Autodesk Fusion 360 part; units mm, degrees
(part 4 of 5)
sketch "Sketch10" plane through (0, 0, 4.8) normal (0, 0, 1) x (-1, 0, 0)
  circle A0 centre (0, 0) radius 3
  line L0 (57.7941, -61.1213) -> (57.7941, -86.8787)
  arc A1 (55.6728, -89) -> (57.7941, -86.8787) centre (56.7335, -87.9393) ccw
  line L1 (55.6728, -89) -> (53.2941, -89)
  line L2 (53.2941, -89) -> (53.2941, -89.8787)
  arc A2 (51.1728, -92) -> (53.2941, -89.8787) centre (52.2335, -90.9393) ccw
  line L3 (51.1728, -92) -> (18.4155, -92)
  arc A3 (16.2941, -89.8787) -> (18.4155, -92) centre (17.3548, -90.9393) ccw
  line L4 (16.2941, -89.8787) -> (16.2941, -89)
  line L5 (16.2941, -89) -> (13.9155, -89)
  arc A4 (11.7941, -86.8787) -> (13.9155, -89) centre (12.8548, -87.9393) ccw
  line L6 (11.7941, -86.8787) -> (11.7941, -61.1213)
  arc A5 (13.9155, -59) -> (11.7941, -61.1213) centre (12.8548, -60.0607) ccw
  line L7 (13.9155, -59) -> (16.2941, -59)
  line L8 (16.2941, -59) -> (16.2941, -58.1213)
  arc A6 (18.4155, -56) -> (16.2941, -58.1213) centre (17.3548, -57.0607) ccw
  line L9 (18.4155, -56) -> (51.1728, -56)
  arc A7 (53.2941, -58.1213) -> (51.1728, -56) centre (52.2335, -57.0607) ccw
  line L10 (53.2941, -58.1213) -> (53.2941, -59)
  line L11 (53.2941, -59) -> (55.6728, -59)
  arc A8 (57.7941, -61.1213) -> (55.6728, -59) centre (56.7335, -60.0607) ccw
  line L12 (51.1728, 56) -> (18.4155, 56)
  arc A9 (16.2941, 58.1213) -> (18.4155, 56) centre (17.3548, 57.0607) ccw
  line L13 (16.2941, 58.1213) -> (16.2941, 59)
  line L14 (16.2941, 59) -> (13.9155, 59)
  arc A10 (11.7941, 61.1213) -> (13.9155, 59) centre (12.8548, 60.0607) ccw
  line L15 (11.7941, 61.1213) -> (11.7941, 86.8787)
  arc A11 (13.9155, 89) -> (11.7941, 86.8787) centre (12.8548, 87.9393) ccw
  line L16 (13.9155, 89) -> (16.2941, 89)
  line L17 (16.2941, 89) -> (16.2941, 89.8787)
  arc A12 (18.4155, 92) -> (16.2941, 89.8787) centre (17.3548, 90.9393) ccw
  line L18 (18.4155, 92) -> (51.1728, 92)
  arc A13 (53.2941, 89.8787) -> (51.1728, 92) centre (52.2335, 90.9393) ccw
  line L19 (53.2941, 89.8787) -> (53.2941, 89)
  line L20 (53.2941, 89) -> (55.6728, 89)
  arc A14 (57.7941, 86.8787) -> (55.6728, 89) centre (56.7335, 87.9393) ccw
  line L21 (57.7941, 86.8787) -> (57.7941, 61.1213)
  arc A15 (55.6728, 59) -> (57.7941, 61.1213) centre (56.7335, 60.0607) ccw
  line L22 (55.6728, 59) -> (53.2941, 59)
  line L23 (53.2941, 59) -> (53.2941, 58.1213)
  arc A16 (51.1728, 56) -> (53.2941, 58.1213) centre (52.2335, 57.0607) ccw
  arc A17 (65.7941, 74.3) -> (67.2941, 72.8) centre (67.2941, 74.3) ccw
  line L24 (65.7941, 74.3) -> (65.7941, 100.26)
  arc A18 (68.1301, 101.5054) -> (65.7941, 100.26) centre (67.2941, 100.26) ccw
  arc A19 (96.3668, 75.223) -> (68.1301, 101.5054) centre (0, 0) ccw
  arc A20 (95.1844, 72.8) -> (96.3668, 75.223) centre (95.1844, 74.3) ccw
  line L25 (95.1844, 72.8) -> (67.2941, 72.8)
  arc A21 (65.7941, -100.26) -> (68.1301, -101.5054) centre (67.2941, -100.26) ccw
  line L26 (65.7941, -100.26) -> (65.7941, -74.3)
  arc A22 (67.2941, -72.8) -> (65.7941, -74.3) centre (67.2941, -74.3) ccw
  line L27 (67.2941, -72.8) -> (95.1844, -72.8)
  arc A23 (96.3668, -75.223) -> (95.1844, -72.8) centre (95.1844, -74.3) ccw
  arc A24 (68.1301, -101.5054) -> (96.3668, -75.223) centre (0, 0) ccw
  circle A25 centre (64.2941, -62.4) radius 1.5
  circle A26 centre (64.2941, 62.4) radius 1.5
  circle A27 centre (97.2941, -62.4) radius 1.5
  circle A28 centre (97.2941, 62.4) radius 1.5
  line L28 (15.4941, 111.4) -> (41.8941, 111.4)
  arc A29 (45.5941, 107.7) -> (41.8941, 111.4) centre (41.8941, 107.7) ccw
  line L29 (45.5941, 107.7) -> (45.5941, 100.7)
  arc A30 (41.8941, 97) -> (45.5941, 100.7) centre (41.8941, 100.7) ccw
  line L30 (41.8941, 97) -> (15.4941, 97)
  arc A31 (11.7941, 100.7) -> (15.4941, 97) centre (15.4941, 100.7) ccw
  line L31 (11.7941, 100.7) -> (11.7941, 107.7)
  arc A32 (15.4941, 111.4) -> (11.7941, 107.7) centre (15.4941, 107.7) ccw
  line L32 (15.4941, -97) -> (41.8941, -97)
  arc A33 (45.5941, -100.7) -> (41.8941, -97) centre (41.8941, -100.7) ccw
  line L33 (45.5941, -100.7) -> (45.5941, -107.7)
  arc A34 (41.8941, -111.4) -> (45.5941, -107.7) centre (41.8941, -107.7) ccw
  line L34 (41.8941, -111.4) -> (15.4941, -111.4)
  arc A35 (11.7941, -107.7) -> (15.4941, -111.4) centre (15.4941, -107.7) ccw
  line L35 (11.7941, -107.7) -> (11.7941, -100.7)
  arc A36 (15.4941, -97) -> (11.7941, -100.7) centre (15.4941, -100.7) ccw
  arc A37 (94.6728, -10) -> (96.7941, -7.8787) centre (95.7335, -8.9393) ccw
  line L36 (94.6728, -10) -> (94.1155, -10)
  arc A38 (91.9941, -7.8787) -> (94.1155, -10) centre (93.0548, -8.9393) ccw
  line L37 (91.9941, -7.8787) -> (91.9941, 7.8787)
  arc A39 (94.1155, 10) -> (91.9941, 7.8787) centre (93.0548, 8.9393) ccw
  line L38 (94.1155, 10) -> (94.6728, 10)
  arc A40 (96.7941, 7.8787) -> (94.6728, 10) centre (95.7335, 8.9393) ccw
  line L39 (96.7941, 7.8787) -> (96.7941, -7.8787)
  circle A41 centre (-94.9024, 87.3758) radius 1.5
  circle A42 centre (123.1209, -38.5) radius 1.5
  circle A43 centre (45.4941, 42.5) radius 1.5
  circle A44 centre (45.4941, -42.5) radius 1.5
  circle A45 centre (123.1209, 38.5) radius 1.5
  circle A46 centre (64.5, -111.7173) radius 1.5
  circle A47 centre (-28.2185, 125.8758) radius 1.5
  circle A48 centre (-94.9024, -87.3758) radius 1.5
  circle A49 centre (-28.2185, -125.8758) radius 1.5
  circle A50 centre (64.5, 111.7173) radius 1.5
  circle A51 centre (-123.5112, -37.2289) radius 1.5
  circle A52 centre (-123.5112, 37.2289) radius 1.5
  arc A53 (-55.2202, 79.8868) -> (-55.9967, 76.9891) centre (-55.6084, 78.438) ccw
  line L40 (-55.2202, 79.8868) -> (-41.5739, 87.7655)
  arc A54 (-38.6762, 86.9891) -> (-41.5739, 87.7655) centre (-40.125, 87.3773) ccw
  line L41 (-38.6762, 86.9891) -> (-38.3975, 86.5064)
  arc A55 (-39.1739, 83.6086) -> (-38.3975, 86.5064) centre (-38.7857, 85.0575) ccw
  line L42 (-39.1739, 83.6086) -> (-52.8202, 75.7299)
  arc A56 (-55.718, 76.5064) -> (-52.8202, 75.7299) centre (-54.2691, 76.1181) ccw
  line L43 (-55.718, 76.5064) -> (-55.9967, 76.9891)
  arc A57 (-11.2762, 39.5309) -> (-14.1739, 40.3073) centre (-12.725, 39.9191) ccw
  line L44 (-11.2762, 39.5309) -> (-10.9975, 39.0482)
  arc A58 (-11.7739, 36.1504) -> (-10.9975, 39.0482) centre (-11.3857, 37.5993) ccw
  line L45 (-11.7739, 36.1504) -> (-25.4202, 28.2717)
  arc A59 (-28.318, 29.0482) -> (-25.4202, 28.2717) centre (-26.8691, 28.66) ccw
  line L46 (-28.318, 29.0482) -> (-28.5967, 29.5309)
  arc A60 (-27.8202, 32.4286) -> (-28.5967, 29.5309) centre (-28.2084, 30.9798) ccw
  line L47 (-27.8202, 32.4286) -> (-14.1739, 40.3073)
  arc A61 (-10.9975, -39.0482) -> (-11.7739, -36.1504) centre (-11.3857, -37.5993) ccw
  line L48 (-10.9975, -39.0482) -> (-11.2762, -39.5309)
  arc A62 (-14.1739, -40.3073) -> (-11.2762, -39.5309) centre (-12.725, -39.9191) ccw
  line L49 (-14.1739, -40.3073) -> (-27.8202, -32.4286)
  arc A63 (-28.5967, -29.5309) -> (-27.8202, -32.4286) centre (-28.2084, -30.9798) ccw
  line L50 (-28.5967, -29.5309) -> (-28.318, -29.0482)
  arc A64 (-25.4202, -28.2717) -> (-28.318, -29.0482) centre (-26.8691, -28.66) ccw
  line L51 (-25.4202, -28.2717) -> (-11.7739, -36.1504)
  arc A65 (-52.8202, -75.7299) -> (-55.718, -76.5064) centre (-54.2691, -76.1181) ccw
  line L52 (-52.8202, -75.7299) -> (-39.1739, -83.6086)
  arc A66 (-38.3975, -86.5064) -> (-39.1739, -83.6086) centre (-38.7857, -85.0575) ccw
  line L53 (-38.3975, -86.5064) -> (-38.6762, -86.9891)
  arc A67 (-41.5739, -87.7655) -> (-38.6762, -86.9891) centre (-40.125, -87.3773) ccw
  line L54 (-41.5739, -87.7655) -> (-55.2202, -79.8868)
  arc A68 (-55.9967, -76.9891) -> (-55.2202, -79.8868) centre (-55.6084, -78.438) ccw
  line L55 (-55.9967, -76.9891) -> (-55.718, -76.5064)
  arc A69 (39.8728, -10) -> (41.9941, -7.8787) centre (40.9335, -8.9393) ccw
  line L56 (39.8728, -10) -> (39.3155, -10)
  arc A70 (37.1941, -7.8787) -> (39.3155, -10) centre (38.2548, -8.9393) ccw
  line L57 (37.1941, -7.8787) -> (37.1941, 7.8787)
  arc A71 (39.3155, 10) -> (37.1941, 7.8787) centre (38.2548, 8.9393) ccw
  line L58 (39.3155, 10) -> (39.8728, 10)
  arc A72 (41.9941, 7.8787) -> (39.8728, 10) centre (40.9335, 8.9393) ccw
  line L59 (41.9941, 7.8787) -> (41.9941, -7.8787)
  line L60 (-42.1213, -25.5) -> (-109.5263, -25.5)
  arc A73 (-109.5263, -25.5) -> (-110.7763, -25.8349) centre (-109.5263, -28) ccw
  line L61 (-110.7763, -25.8349) -> (-125.9451, -34.5927)
  arc A74 (-125.9451, -34.5927) -> (-127.0931, -37.4646) centre (-124.6951, -36.7577) ccw
  arc A75 (-127.0931, -37.4646) -> (-89.0244, -98.1371) centre (0, 0) ccw
  arc A76 (-89.0244, -98.1371) -> (-85.1797, -97.5355) centre (-87.3447, -96.2855) ccw
  line L62 (-85.1797, -97.5355) -> (-74.6084, -79.2255)
  arc A77 (-71.7106, -78.449) -> (-74.6084, -79.2255) centre (-73.1595, -78.8372) ccw
  line L63 (-71.7106, -78.449) -> (-32.0836, -101.3277)
  arc A78 (-31.3071, -104.2255) -> (-32.0836, -101.3277) centre (-31.6953, -102.7766) ccw
  line L64 (-31.3071, -104.2255) -> (-41.8784, -122.5355)
  arc A79 (-41.8784, -122.5355) -> (-40.477, -126.166) centre (-39.7133, -123.7855) ccw
  arc A80 (-40.477, -126.166) -> (129.5015, -28.0288) centre (0, 0) ccw
  arc A81 (129.5015, -28.0288) -> (127.0581, -25) centre (127.0581, -27.5) ccw
  line L65 (127.0581, -25) -> (105.9155, -25)
  arc A82 (103.7941, -22.8787) -> (105.9155, -25) centre (104.8548, -23.9393) ccw
  line L66 (103.7941, -22.8787) -> (103.7941, 22.8787)
  arc A83 (105.9155, 25) -> (103.7941, 22.8787) centre (104.8548, 23.9393) ccw
  line L67 (105.9155, 25) -> (127.0581, 25)
  arc A84 (127.0581, 25) -> (129.5015, 28.0288) centre (127.0581, 27.5) ccw
  arc A85 (129.5015, 28.0288) -> (-40.477, 126.166) centre (0, 0) ccw
  arc A86 (-40.477, 126.166) -> (-41.8784, 122.5355) centre (-39.7133, 123.7855) ccw
  line L68 (-41.8784, 122.5355) -> (-31.3071, 104.2255)
  arc A87 (-32.0836, 101.3277) -> (-31.3071, 104.2255) centre (-31.6953, 102.7766) ccw
  line L69 (-32.0836, 101.3277) -> (-71.7106, 78.449)
  arc A88 (-74.6084, 79.2255) -> (-71.7106, 78.449) centre (-73.1595, 78.8372) ccw
  line L70 (-74.6084, 79.2255) -> (-85.1797, 97.5355)
  arc A89 (-85.1797, 97.5355) -> (-89.0244, 98.1371) centre (-87.3447, 96.2855) ccw
  arc A90 (-89.0244, 98.1371) -> (-127.0931, 37.4646) centre (0, 0) ccw
  arc A91 (-127.0931, 37.4646) -> (-125.9451, 34.5927) centre (-124.6951, 36.7577) ccw
  line L71 (-125.9451, 34.5927) -> (-110.7763, 25.8349)
  arc A92 (-110.7763, 25.8349) -> (-109.5263, 25.5) centre (-109.5263, 28) ccw
  line L72 (-109.5263, 25.5) -> (-42.1213, 25.5)
  arc A93 (-40, 23.3787) -> (-42.1213, 25.5) centre (-41.0607, 24.4393) ccw
  line L73 (-40, 23.3787) -> (-40, 20.8)
  arc A94 (-40, 20.8) -> (-37.5, 18.3) centre (-37.5, 20.8) ccw
  line L74 (-37.5, 18.3) -> (-34.1213, 18.3)
  arc A95 (-32, 16.1787) -> (-34.1213, 18.3) centre (-33.0607, 17.2393) ccw
  line L75 (-32, 16.1787) -> (-32, -16.1787)
  arc A96 (-34.1213, -18.3) -> (-32, -16.1787) centre (-33.0607, -17.2393) ccw
  line L76 (-34.1213, -18.3) -> (-37.5, -18.3)
  arc A97 (-37.5, -18.3) -> (-40, -20.8) centre (-37.5, -20.8) ccw
  line L77 (-40, -20.8) -> (-40, -23.3787)
  arc A98 (-42.1213, -25.5) -> (-40, -23.3787) centre (-41.0607, -24.4393) ccw
  line L78 (-42.1213, 25.5) -> (-109.5263, 25.5)
  line L79 (-42.1213, -25.5) -> (-109.5263, -25.5)
  arc A99 (-127.0931, -37.4646) -> (-89.0244, -98.1371) centre (0, 0) ccw
  arc A100 (-89.0244, 98.1371) -> (-127.0931, 37.4646) centre (0, 0) ccw
  line L80 (-25.6319, 7.5958) -> (-67.8319, 80.6884)
  line L81 (-25.6319, -7.5958) -> (-67.8319, -80.6884)
  circle A101 centre (-53.2894, 35.5) radius 1.5
  circle A102 centre (-100, 35.5) radius 1.5
  line L82 (-130.0231, 25.5) -> (-40, 25.5)
  line L83 (-100, 25.5) -> (-100, -25.5) construction
  line L84 (-40, 25.5) -> (-40, -25.5) construction
  line L85 (-100, 25.5) -> (-100, 35.5) construction
  circle A103 centre (-53.2894, -35.5) radius 1.5
  circle A104 centre (-100, -35.5) radius 1.5
  line L86 (-100, -25.5) -> (-100, -35.5) construction
  line L87 (-103, 28.5) -> (-103, 35.5)
  line L88 (-100, 38.5) -> (-48.1666, 38.5)
  line L89 (0, 0) -> (-44.1633, 38.5) construction
  line L90 (-47.1809, 41.1307) -> (-97.2023, 84.7376)
  line L91 (-85.1797, 97.5355) -> (-74.6084, 79.2255)
  line L92 (-103, 25.5) -> (-103, 28.5) construction
  arc A105 (-100, 25.5) -> (-103, 28.5) centre (-100, 28.5) ccw construction
  arc A106 (-103, 28.5) -> (-100, 25.5) centre (-100, 28.5) ccw
  arc A107 (-48.1666, 38.5) -> (-47.1809, 41.1307) centre (-48.1666, 40) ccw
  arc A108 (-100, 38.5) -> (-103, 35.5) centre (-100, 35.5) ccw
  arc A109 (-40.477, 126.166) -> (-40.477, -126.166) centre (0, 0) ccw
  line L93 (-97.2023, 84.7376) -> (-99.8764, 87.0687) construction
  arc A110 (-97.2023, 84.7376) -> (-97.4773, 89.7465) centre (-94.9024, 87.3758) ccw construction
  arc A111 (-97.4773, 89.7465) -> (-97.2023, 84.7376) centre (-94.9024, 87.3758) ccw
  line L94 (0, 0) -> (-44.1633, -38.5) construction
  line L95 (-48.1666, -38.5) -> (-100, -38.5)
  line L96 (-103, -35.5) -> (-103, -28.5)
  line L97 (-47.1809, -41.1307) -> (-97.2023, -84.7376)
  arc A112 (-47.1809, -41.1307) -> (-48.1666, -38.5) centre (-48.1666, -40) ccw
  arc A113 (-103, -35.5) -> (-100, -38.5) centre (-100, -35.5) ccw
  arc A114 (-97.4773, -89.7465) -> (-97.2023, -84.7376) centre (-94.9024, -87.3758) ccw construction
  arc A115 (-97.2023, -84.7376) -> (-97.4773, -89.7465) centre (-94.9024, -87.3758) ccw
  line L98 (-97.2023, -84.7376) -> (-99.8764, -87.0687) construction
  line L99 (-40, -25.5) -> (-130.0231, -25.5)
  arc A116 (-100, -31.5) -> (-100, -25.5) centre (-100, -28.5) ccw construction
  arc A117 (-100, -25.5) -> (-103, -28.5) centre (-100, -28.5) ccw
  arc A118 (-103, -28.5) -> (-100, -31.5) centre (-100, -28.5) ccw construction
  line L100 (-103, -28.5) -> (-103, -25.5) construction
  point P0 (-94.9024, 87.3758)
  point P1 (-94.9024, -87.3758)
  dimension "d371" = 3
  dimension "d372" = 3
  dimension "d373" = 10
  dimension "d374" = 10
  dimension "d375" = 10
  dimension "d376" = 60
  dimension "d377" = 3
  dimension "d378" = 3
  dimension "d379" = 10
  dimension "d380" = 10
  dimension "d381" = 10
  dimension "d383" = 3
  dimension "d384" = 3
  dimension "d385" = 6
  dimension "d386" = 1.5
  dimension "d387" = 3
  dimension "d388" = 7
  dimension "d389" = 3.5
  dimension "d390" = 3
  dimension "d391" = 3
  dimension "d392" = 3.5
  dimension "d393" = 1.5
  dimension "d394" = 3
  dimension "d395" = 3
  constraint coincident L82 L83.start
  constraint coincident L79 L83.end
  constraint perpendicular L79 L83
  constraint coincident A102.centre L85.end
  constraint vertical L85
  constraint coincident A104.centre L86.end
  constraint vertical L86
  constraint coincident L82 L92.start
  constraint perpendicular L82 L87
  constraint perpendicular L85 L88
  constraint coincident A0.centre A19.centre
  constraint coincident A100 L93.end
  constraint parallel L89 L90
  constraint tangent L87 A105
  constraint tangent L82 A105
  constraint perpendicular L82 L92
  constraint coincident L72 L83.start
  constraint concentric A105 A106
  constraint coincident L89.end L90
  constraint coincident L89.end L88
  constraint tangent L90 A107
  constraint tangent L88 A107
  constraint tangent L88 A108
  constraint tangent L87 A108
  constraint tangent L90 A110
  constraint tangent A109 A110
  constraint parallel L89 L93
  constraint coincident A90 A110.end
  constraint concentric A110 A111
  constraint coincident A99 L98.end
  constraint horizontal L95
  constraint coincident L79 L100.end
  constraint perpendicular L79 L96
  constraint coincident L94.end L97
  constraint coincident L94.end L95
  constraint tangent L97 A112
  constraint tangent L95 A112
  constraint tangent L95 A113
  constraint tangent L96 A113
  constraint coincident P1 A48.centre
  constraint tangent L97 A114
  constraint coincident A75 A114.start
  constraint concentric A114 A115
  constraint coincident L94.end L98
  constraint tangent L96 A116
  constraint tangent L99 A116
  constraint coincident L60 L83.end
  constraint concentric A116 A117
  constraint coincident L86 A116.start
  constraint concentric A116 A118
  constraint perpendicular L79 L100
  measures "d371" diameter of A101
  measures "d372" diameter of A102
  measures "d373" distance of L80 A101.centre
  measures "d374" distance of A101.centre L82
  measures "d375" distance of L78 A102.centre
  measures "d376" distance of L83 L84
  measures "d377" diameter of A103
  measures "d378" diameter of A104
  measures "d379" distance of L79 A104.centre
  measures "d380" distance of L79 A103.centre
  measures "d381" distance of L81 A103.centre
  measures "d383" distance of A102.centre L88
  measures "d384" distance of A102.centre L87
  measures "d385" diameter of A105
  measures "d386" radius of A107
  measures "d387" radius of A108
  measures "d388" diameter of A110
  measures "d389" distance of L90 P0
  measures "d390" distance of A104.centre L96
  measures "d391" distance of A104.centre L95
  measures "d392" distance of L94 P1
  measures "d393" radius of A112
  measures "d394" radius of A113
  measures "d395" radius of A117
extrude "Extrude13" cut sketch "Sketch10" against normal through all contours L60 A73 L61 A74 A75 L79 A99 A109 L95 L96 L97 A112 A113 A115 L99 A117 | A90 A91 L71 A92 L72 L78 A100 L82 L87 L88 L90 A106 A107 A108 A109 A111 | A101 | A102 | A103 | A104
sketch "Sketch11" plane through (0, 0, 4.8) normal (0, 0, 1) x (-1, 0, 0)
  arc A0 (-97.4773, 89.7465) -> (-97.2023, 84.7376) centre (-94.9024, 87.3758) ccw
  line L0 (-97.2023, 84.7376) -> (-47.1809, 41.1307)
  arc A1 (-48.1666, 38.5) -> (-47.1809, 41.1307) centre (-48.1666, 40) ccw
  line L1 (-48.1666, 38.5) -> (-100, 38.5)
  arc A2 (-100, 38.5) -> (-103, 35.5) centre (-100, 35.5) ccw
  line L2 (-103, 35.5) -> (-103, 28.5)
  arc A3 (-103, 28.5) -> (-100, 25.5) centre (-100, 28.5) ccw
  line L3 (-100, 25.5) -> (-42.1213, 25.5)
  arc A4 (-40, 23.3787) -> (-42.1213, 25.5) centre (-41.0607, 24.4393) ccw
  line L4 (-40, 23.3787) -> (-40, 20.8)
  arc A5 (-40, 20.8) -> (-37.5, 18.3) centre (-37.5, 20.8) ccw
  line L5 (-37.5, 18.3) -> (-34.1213, 18.3)
  arc A6 (-32, 16.1787) -> (-34.1213, 18.3) centre (-33.0607, 17.2393) ccw
  line L6 (-32, 16.1787) -> (-32, -16.1787)
  arc A7 (-34.1213, -18.3) -> (-32, -16.1787) centre (-33.0607, -17.2393) ccw
  line L7 (-34.1213, -18.3) -> (-37.5, -18.3)
  arc A8 (-37.5, -18.3) -> (-40, -20.8) centre (-37.5, -20.8) ccw
  line L8 (-40, -20.8) -> (-40, -23.3787)
  arc A9 (-42.1213, -25.5) -> (-40, -23.3787) centre (-41.0607, -24.4393) ccw
  line L9 (-42.1213, -25.5) -> (-100, -25.5)
  arc A10 (-100, -25.5) -> (-103, -28.5) centre (-100, -28.5) ccw
  line L10 (-103, -28.5) -> (-103, -35.5)
  arc A11 (-103, -35.5) -> (-100, -38.5) centre (-100, -35.5) ccw
  line L11 (-100, -38.5) -> (-48.1666, -38.5)
  arc A12 (-47.1809, -41.1307) -> (-48.1666, -38.5) centre (-48.1666, -40) ccw
  line L12 (-47.1809, -41.1307) -> (-97.2023, -84.7376)
  arc A13 (-97.2023, -84.7376) -> (-97.4773, -89.7465) centre (-94.9024, -87.3758) ccw
  arc A14 (-97.4773, -89.7465) -> (-89.0244, -98.1371) centre (0, 0) ccw
  arc A15 (-89.0244, -98.1371) -> (-85.1797, -97.5355) centre (-87.3447, -96.2855) ccw
  line L13 (-85.1797, -97.5355) -> (-74.6084, -79.2255)
  arc A16 (-71.7106, -78.449) -> (-74.6084, -79.2255) centre (-73.1595, -78.8372) ccw
  line L14 (-71.7106, -78.449) -> (-32.0836, -101.3277)
  arc A17 (-31.3071, -104.2255) -> (-32.0836, -101.3277) centre (-31.6953, -102.7766) ccw
  line L15 (-31.3071, -104.2255) -> (-41.8784, -122.5355)
  arc A18 (-41.8784, -122.5355) -> (-40.477, -126.166) centre (-39.7133, -123.7855) ccw
  arc A19 (-40.477, -126.166) -> (129.5015, -28.0288) centre (0, 0) ccw
  arc A20 (129.5015, -28.0288) -> (127.0581, -25) centre (127.0581, -27.5) ccw
  line L16 (127.0581, -25) -> (105.9155, -25)
  arc A21 (103.7941, -22.8787) -> (105.9155, -25) centre (104.8548, -23.9393) ccw
  line L17 (103.7941, -22.8787) -> (103.7941, 22.8787)
  arc A22 (105.9155, 25) -> (103.7941, 22.8787) centre (104.8548, 23.9393) ccw
  line L18 (105.9155, 25) -> (127.0581, 25)
  arc A23 (127.0581, 25) -> (129.5015, 28.0288) centre (127.0581, 27.5) ccw
  arc A24 (129.5015, 28.0288) -> (-40.477, 126.166) centre (0, 0) ccw
  arc A25 (-40.477, 126.166) -> (-41.8784, 122.5355) centre (-39.7133, 123.7855) ccw
  line L19 (-41.8784, 122.5355) -> (-31.3071, 104.2255)
  arc A26 (-32.0836, 101.3277) -> (-31.3071, 104.2255) centre (-31.6953, 102.7766) ccw
  line L20 (-32.0836, 101.3277) -> (-71.7106, 78.449)
  arc A27 (-74.6084, 79.2255) -> (-71.7106, 78.449) centre (-73.1595, 78.8372) ccw
  line L21 (-74.6084, 79.2255) -> (-85.1797, 97.5355)
  arc A28 (-85.1797, 97.5355) -> (-89.0244, 98.1371) centre (-87.3447, 96.2855) ccw
  arc A29 (-89.0244, 98.1371) -> (-97.4773, 89.7465) centre (0, 0) ccw
  circle A30 centre (-28.2185, 125.8758) radius 1.5
  arc A31 (-52.8202, -75.7299) -> (-55.718, -76.5064) centre (-54.2691, -76.1181) ccw
  line L22 (-52.8202, -75.7299) -> (-39.1739, -83.6086)
  arc A32 (-38.3975, -86.5064) -> (-39.1739, -83.6086) centre (-38.7857, -85.0575) ccw
  line L23 (-38.3975, -86.5064) -> (-38.6762, -86.9891)
  arc A33 (-41.5739, -87.7655) -> (-38.6762, -86.9891) centre (-40.125, -87.3773) ccw
  line L24 (-41.5739, -87.7655) -> (-55.2202, -79.8868)
  arc A34 (-55.9967, -76.9891) -> (-55.2202, -79.8868) centre (-55.6084, -78.438) ccw
  line L25 (-55.9967, -76.9891) -> (-55.718, -76.5064)
  circle A35 centre (123.1209, -38.5) radius 1.5
  arc A36 (-11.2762, 39.5309) -> (-14.1739, 40.3073) centre (-12.725, 39.9191) ccw
  line L26 (-11.2762, 39.5309) -> (-10.9975, 39.0482)
  arc A37 (-11.7739, 36.1504) -> (-10.9975, 39.0482) centre (-11.3857, 37.5993) ccw
  line L27 (-11.7739, 36.1504) -> (-25.4202, 28.2717)
  arc A38 (-28.318, 29.0482) -> (-25.4202, 28.2717) centre (-26.8691, 28.66) ccw
  line L28 (-28.318, 29.0482) -> (-28.5967, 29.5309)
  arc A39 (-27.8202, 32.4286) -> (-28.5967, 29.5309) centre (-28.2084, 30.9798) ccw
  line L29 (-27.8202, 32.4286) -> (-14.1739, 40.3073)
  arc A40 (-10.9975, -39.0482) -> (-11.7739, -36.1504) centre (-11.3857, -37.5993) ccw
  line L30 (-10.9975, -39.0482) -> (-11.2762, -39.5309)
  arc A41 (-14.1739, -40.3073) -> (-11.2762, -39.5309) centre (-12.725, -39.9191) ccw
  line L31 (-14.1739, -40.3073) -> (-27.8202, -32.4286)
  arc A42 (-28.5967, -29.5309) -> (-27.8202, -32.4286) centre (-28.2084, -30.9798) ccw
  line L32 (-28.5967, -29.5309) -> (-28.318, -29.0482)
  arc A43 (-25.4202, -28.2717) -> (-28.318, -29.0482) centre (-26.8691, -28.66) ccw
  line L33 (-25.4202, -28.2717) -> (-11.7739, -36.1504)
  circle A44 centre (64.5, -111.7173) radius 1.5
  arc A45 (39.8728, -10) -> (41.9941, -7.8787) centre (40.9335, -8.9393) ccw
  line L34 (39.8728, -10) -> (39.3155, -10)
  arc A46 (37.1941, -7.8787) -> (39.3155, -10) centre (38.2548, -8.9393) ccw
  line L35 (37.1941, -7.8787) -> (37.1941, 7.8787)
  arc A47 (39.3155, 10) -> (37.1941, 7.8787) centre (38.2548, 8.9393) ccw
  line L36 (39.3155, 10) -> (39.8728, 10)
  arc A48 (41.9941, 7.8787) -> (39.8728, 10) centre (40.9335, 8.9393) ccw
  line L37 (41.9941, 7.8787) -> (41.9941, -7.8787)
  circle A49 centre (-94.9024, -87.3758) radius 1.5
  circle A50 centre (-28.2185, -125.8758) radius 1.5
  circle A51 centre (64.5, 111.7173) radius 1.5
  arc A52 (-55.2202, 79.8868) -> (-55.9967, 76.9891) centre (-55.6084, 78.438) ccw
  line L38 (-55.2202, 79.8868) -> (-41.5739, 87.7655)
  arc A53 (-38.6762, 86.9891) -> (-41.5739, 87.7655) centre (-40.125, 87.3773) ccw
  line L39 (-38.6762, 86.9891) -> (-38.3975, 86.5064)
  arc A54 (-39.1739, 83.6086) -> (-38.3975, 86.5064) centre (-38.7857, 85.0575) ccw
  line L40 (-39.1739, 83.6086) -> (-52.8202, 75.7299)
  arc A55 (-55.718, 76.5064) -> (-52.8202, 75.7299) centre (-54.2691, 76.1181) ccw
  line L41 (-55.718, 76.5064) -> (-55.9967, 76.9891)
  circle A56 centre (123.1209, 38.5) radius 1.5
  circle A57 centre (45.4941, 42.5) radius 1.5
  circle A58 centre (-94.9024, 87.3758) radius 1.5
  arc A59 (94.6728, -10) -> (96.7941, -7.8787) centre (95.7335, -8.9393) ccw
  line L42 (94.6728, -10) -> (94.1155, -10)
  arc A60 (91.9941, -7.8787) -> (94.1155, -10) centre (93.0548, -8.9393) ccw
  line L43 (91.9941, -7.8787) -> (91.9941, 7.8787)
  arc A61 (94.1155, 10) -> (91.9941, 7.8787) centre (93.0548, 8.9393) ccw
  line L44 (94.1155, 10) -> (94.6728, 10)
  arc A62 (96.7941, 7.8787) -> (94.6728, 10) centre (95.7335, 8.9393) ccw
  line L45 (96.7941, 7.8787) -> (96.7941, -7.8787)
  circle A63 centre (45.4941, -42.5) radius 1.5
  line L46 (15.4941, -97) -> (41.8941, -97)
  arc A64 (45.5941, -100.7) -> (41.8941, -97) centre (41.8941, -100.7) ccw
  line L47 (45.5941, -100.7) -> (45.5941, -107.7)
  arc A65 (41.8941, -111.4) -> (45.5941, -107.7) centre (41.8941, -107.7) ccw
  line L48 (41.8941, -111.4) -> (15.4941, -111.4)
  arc A66 (11.7941, -107.7) -> (15.4941, -111.4) centre (15.4941, -107.7) ccw
  line L49 (11.7941, -107.7) -> (11.7941, -100.7)
  arc A67 (15.4941, -97) -> (11.7941, -100.7) centre (15.4941, -100.7) ccw
  line L50 (15.4941, 111.4) -> (41.8941, 111.4)
  arc A68 (45.5941, 107.7) -> (41.8941, 111.4) centre (41.8941, 107.7) ccw
  line L51 (45.5941, 107.7) -> (45.5941, 100.7)
  arc A69 (41.8941, 97) -> (45.5941, 100.7) centre (41.8941, 100.7) ccw
  line L52 (41.8941, 97) -> (15.4941, 97)
  arc A70 (11.7941, 100.7) -> (15.4941, 97) centre (15.4941, 100.7) ccw
  line L53 (11.7941, 100.7) -> (11.7941, 107.7)
  arc A71 (15.4941, 111.4) -> (11.7941, 107.7) centre (15.4941, 107.7) ccw
  circle A72 centre (97.2941, 62.4) radius 1.5
  circle A73 centre (97.2941, -62.4) radius 1.5
  circle A74 centre (64.2941, 62.4) radius 1.5
  circle A75 centre (64.2941, -62.4) radius 1.5
  arc A76 (65.7941, -100.26) -> (68.1301, -101.5054) centre (67.2941, -100.26) ccw
  line L54 (65.7941, -100.26) -> (65.7941, -74.3)
  arc A77 (67.2941, -72.8) -> (65.7941, -74.3) centre (67.2941, -74.3) ccw
  line L55 (67.2941, -72.8) -> (95.1844, -72.8)
  arc A78 (96.3668, -75.223) -> (95.1844, -72.8) centre (95.1844, -74.3) ccw
  arc A79 (68.1301, -101.5054) -> (96.3668, -75.223) centre (0, 0) ccw
  arc A80 (65.7941, 74.3) -> (67.2941, 72.8) centre (67.2941, 74.3) ccw
  line L56 (65.7941, 74.3) -> (65.7941, 100.26)
  arc A81 (68.1301, 101.5054) -> (65.7941, 100.26) centre (67.2941, 100.26) ccw
  arc A82 (96.3668, 75.223) -> (68.1301, 101.5054) centre (0, 0) ccw
  arc A83 (95.1844, 72.8) -> (96.3668, 75.223) centre (95.1844, 74.3) ccw
  line L57 (95.1844, 72.8) -> (67.2941, 72.8)
  line L58 (51.1728, 56) -> (18.4155, 56)
  arc A84 (16.2941, 58.1213) -> (18.4155, 56) centre (17.3548, 57.0607) ccw
  line L59 (16.2941, 58.1213) -> (16.2941, 59)
  line L60 (16.2941, 59) -> (13.9155, 59)
  arc A85 (11.7941, 61.1213) -> (13.9155, 59) centre (12.8548, 60.0607) ccw
  line L61 (11.7941, 61.1213) -> (11.7941, 86.8787)
  arc A86 (13.9155, 89) -> (11.7941, 86.8787) centre (12.8548, 87.9393) ccw
  line L62 (13.9155, 89) -> (16.2941, 89)
  line L63 (16.2941, 89) -> (16.2941, 89.8787)
  arc A87 (18.4155, 92) -> (16.2941, 89.8787) centre (17.3548, 90.9393) ccw
  line L64 (18.4155, 92) -> (51.1728, 92)
  arc A88 (53.2941, 89.8787) -> (51.1728, 92) centre (52.2335, 90.9393) ccw
  line L65 (53.2941, 89.8787) -> (53.2941, 89)
  line L66 (53.2941, 89) -> (55.6728, 89)
  arc A89 (57.7941, 86.8787) -> (55.6728, 89) centre (56.7335, 87.9393) ccw
  line L67 (57.7941, 86.8787) -> (57.7941, 61.1213)
  arc A90 (55.6728, 59) -> (57.7941, 61.1213) centre (56.7335, 60.0607) ccw
  line L68 (55.6728, 59) -> (53.2941, 59)
  line L69 (53.2941, 59) -> (53.2941, 58.1213)
  arc A91 (51.1728, 56) -> (53.2941, 58.1213) centre (52.2335, 57.0607) ccw
  line L70 (57.7941, -61.1213) -> (57.7941, -86.8787)
  arc A92 (55.6728, -89) -> (57.7941, -86.8787) centre (56.7335, -87.9393) ccw
  line L71 (55.6728, -89) -> (53.2941, -89)
  line L72 (53.2941, -89) -> (53.2941, -89.8787)
  arc A93 (51.1728, -92) -> (53.2941, -89.8787) centre (52.2335, -90.9393) ccw
  line L73 (51.1728, -92) -> (18.4155, -92)
  arc A94 (16.2941, -89.8787) -> (18.4155, -92) centre (17.3548, -90.9393) ccw
  line L74 (16.2941, -89.8787) -> (16.2941, -89)
  line L75 (16.2941, -89) -> (13.9155, -89)
  arc A95 (11.7941, -86.8787) -> (13.9155, -89) centre (12.8548, -87.9393) ccw
  line L76 (11.7941, -86.8787) -> (11.7941, -61.1213)
  arc A96 (13.9155, -59) -> (11.7941, -61.1213) centre (12.8548, -60.0607) ccw
  line L77 (13.9155, -59) -> (16.2941, -59)
  line L78 (16.2941, -59) -> (16.2941, -58.1213)
  arc A97 (18.4155, -56) -> (16.2941, -58.1213) centre (17.3548, -57.0607) ccw
  line L79 (18.4155, -56) -> (51.1728, -56)
  arc A98 (53.2941, -58.1213) -> (51.1728, -56) centre (52.2335, -57.0607) ccw
  line L80 (53.2941, -58.1213) -> (53.2941, -59)
  line L81 (53.2941, -59) -> (55.6728, -59)
  arc A99 (57.7941, -61.1213) -> (55.6728, -59) centre (56.7335, -60.0607) ccw
  circle A100 centre (0, 0) radius 3
  circle A101 centre (-100, 35.5) radius 1.5
  circle A102 centre (-53.2894, -35.5) radius 1.5
  circle A103 centre (-53.2894, 35.5) radius 1.5
  circle A104 centre (-100, -35.5) radius 1.5
  line L82 (11.7941, 100.7) -> (11.7941, 107.7)
  line L83 (11.7941, 104.2) -> (1.7941, 104.2) construction
  circle A105 centre (1.7941, 104.2) radius 5.5
  circle A106 centre (1.7941, 104.2) radius 6.1
  point P0 (11.7941, 104.2)
  dimension "d397" = 10
  dimension "d398" = 11
  dimension "d399" = 12.2
  constraint midpoint L82 P0
  constraint coincident P0 L83.start
  constraint perpendicular L53 L83
  constraint coincident L83.end A105.centre
  constraint concentric A105 A106
  measures "d397" distance of P0 L83.end
  measures "d398" diameter of A105
  measures "d399" diameter of A106
extrude "Extrude14" cut sketch "Sketch11" against normal through all contours A105
extrude "Extrude15" cut sketch "Sketch11" against normal blind 2 contours A106
sketch "Sketch12" plane through (0, 0, 4.8) normal (0, 0, 1) x (-1, 0, 0)
  circle A0 centre (1.7941, 104.2) radius 6.1
  arc A1 (-97.4773, 89.7465) -> (-97.2023, 84.7376) centre (-94.9024, 87.3758) ccw
  line L0 (-97.2023, 84.7376) -> (-47.1809, 41.1307)
  arc A2 (-48.1666, 38.5) -> (-47.1809, 41.1307) centre (-48.1666, 40) ccw
  line L1 (-48.1666, 38.5) -> (-100, 38.5)
  arc A3 (-100, 38.5) -> (-103, 35.5) centre (-100, 35.5) ccw
  line L2 (-103, 35.5) -> (-103, 28.5)
  arc A4 (-103, 28.5) -> (-100, 25.5) centre (-100, 28.5) ccw
  line L3 (-100, 25.5) -> (-42.1213, 25.5)
  arc A5 (-40, 23.3787) -> (-42.1213, 25.5) centre (-41.0607, 24.4393) ccw
  line L4 (-40, 23.3787) -> (-40, 20.8)
  arc A6 (-40, 20.8) -> (-37.5, 18.3) centre (-37.5, 20.8) ccw
  line L5 (-37.5, 18.3) -> (-34.1213, 18.3)
  arc A7 (-32, 16.1787) -> (-34.1213, 18.3) centre (-33.0607, 17.2393) ccw
  line L6 (-32, 16.1787) -> (-32, -16.1787)
  arc A8 (-34.1213, -18.3) -> (-32, -16.1787) centre (-33.0607, -17.2393) ccw
  line L7 (-34.1213, -18.3) -> (-37.5, -18.3)
  arc A9 (-37.5, -18.3) -> (-40, -20.8) centre (-37.5, -20.8) ccw
  line L8 (-40, -20.8) -> (-40, -23.3787)
  arc A10 (-42.1213, -25.5) -> (-40, -23.3787) centre (-41.0607, -24.4393) ccw
  line L9 (-42.1213, -25.5) -> (-100, -25.5)
  arc A11 (-100, -25.5) -> (-103, -28.5) centre (-100, -28.5) ccw
  line L10 (-103, -28.5) -> (-103, -35.5)
  arc A12 (-103, -35.5) -> (-100, -38.5) centre (-100, -35.5) ccw
  line L11 (-100, -38.5) -> (-48.1666, -38.5)
  arc A13 (-47.1809, -41.1307) -> (-48.1666, -38.5) centre (-48.1666, -40) ccw
  line L12 (-47.1809, -41.1307) -> (-97.2023, -84.7376)
  arc A14 (-97.2023, -84.7376) -> (-97.4773, -89.7465) centre (-94.9024, -87.3758) ccw
  arc A15 (-97.4773, -89.7465) -> (-89.0244, -98.1371) centre (0, 0) ccw
  arc A16 (-89.0244, -98.1371) -> (-85.1797, -97.5355) centre (-87.3447, -96.2855) ccw
  line L13 (-85.1797, -97.5355) -> (-74.6084, -79.2255)
  arc A17 (-71.7106, -78.449) -> (-74.6084, -79.2255) centre (-73.1595, -78.8372) ccw
  line L14 (-71.7106, -78.449) -> (-32.0836, -101.3277)
  arc A18 (-31.3071, -104.2255) -> (-32.0836, -101.3277) centre (-31.6953, -102.7766) ccw
  line L15 (-31.3071, -104.2255) -> (-41.8784, -122.5355)
  arc A19 (-41.8784, -122.5355) -> (-40.477, -126.166) centre (-39.7133, -123.7855) ccw
  arc A20 (-40.477, -126.166) -> (129.5015, -28.0288) centre (0, 0) ccw
  arc A21 (129.5015, -28.0288) -> (127.0581, -25) centre (127.0581, -27.5) ccw
  line L16 (127.0581, -25) -> (105.9155, -25)
  arc A22 (103.7941, -22.8787) -> (105.9155, -25) centre (104.8548, -23.9393) ccw
  line L17 (103.7941, -22.8787) -> (103.7941, 22.8787)
  arc A23 (105.9155, 25) -> (103.7941, 22.8787) centre (104.8548, 23.9393) ccw
  line L18 (105.9155, 25) -> (127.0581, 25)
  arc A24 (127.0581, 25) -> (129.5015, 28.0288) centre (127.0581, 27.5) ccw
  arc A25 (129.5015, 28.0288) -> (-40.477, 126.166) centre (0, 0) ccw
  arc A26 (-40.477, 126.166) -> (-41.8784, 122.5355) centre (-39.7133, 123.7855) ccw
  line L19 (-41.8784, 122.5355) -> (-31.3071, 104.2255)
  arc A27 (-32.0836, 101.3277) -> (-31.3071, 104.2255) centre (-31.6953, 102.7766) ccw
  line L20 (-32.0836, 101.3277) -> (-71.7106, 78.449)
  arc A28 (-74.6084, 79.2255) -> (-71.7106, 78.449) centre (-73.1595, 78.8372) ccw
  line L21 (-74.6084, 79.2255) -> (-85.1797, 97.5355)
  arc A29 (-85.1797, 97.5355) -> (-89.0244, 98.1371) centre (-87.3447, 96.2855) ccw
  arc A30 (-89.0244, 98.1371) -> (-97.4773, 89.7465) centre (0, 0) ccw
  circle A31 centre (-28.2185, 125.8758) radius 1.5
  arc A32 (-52.8202, -75.7299) -> (-55.718, -76.5064) centre (-54.2691, -76.1181) ccw
  line L22 (-52.8202, -75.7299) -> (-39.1739, -83.6086)
  arc A33 (-38.3975, -86.5064) -> (-39.1739, -83.6086) centre (-38.7857, -85.0575) ccw
  line L23 (-38.3975, -86.5064) -> (-38.6762, -86.9891)
  arc A34 (-41.5739, -87.7655) -> (-38.6762, -86.9891) centre (-40.125, -87.3773) ccw
  line L24 (-41.5739, -87.7655) -> (-55.2202, -79.8868)
  arc A35 (-55.9967, -76.9891) -> (-55.2202, -79.8868) centre (-55.6084, -78.438) ccw
  line L25 (-55.9967, -76.9891) -> (-55.718, -76.5064)
  circle A36 centre (123.1209, -38.5) radius 1.5
  arc A37 (-11.2762, 39.5309) -> (-14.1739, 40.3073) centre (-12.725, 39.9191) ccw
  line L26 (-11.2762, 39.5309) -> (-10.9975, 39.0482)
  arc A38 (-11.7739, 36.1504) -> (-10.9975, 39.0482) centre (-11.3857, 37.5993) ccw
  line L27 (-11.7739, 36.1504) -> (-25.4202, 28.2717)
  arc A39 (-28.318, 29.0482) -> (-25.4202, 28.2717) centre (-26.8691, 28.66) ccw
  line L28 (-28.318, 29.0482) -> (-28.5967, 29.5309)
  arc A40 (-27.8202, 32.4286) -> (-28.5967, 29.5309) centre (-28.2084, 30.9798) ccw
  line L29 (-27.8202, 32.4286) -> (-14.1739, 40.3073)
  arc A41 (-10.9975, -39.0482) -> (-11.7739, -36.1504) centre (-11.3857, -37.5993) ccw
  line L30 (-10.9975, -39.0482) -> (-11.2762, -39.5309)
  arc A42 (-14.1739, -40.3073) -> (-11.2762, -39.5309) centre (-12.725, -39.9191) ccw
  line L31 (-14.1739, -40.3073) -> (-27.8202, -32.4286)
  arc A43 (-28.5967, -29.5309) -> (-27.8202, -32.4286) centre (-28.2084, -30.9798) ccw
  line L32 (-28.5967, -29.5309) -> (-28.318, -29.0482)
  arc A44 (-25.4202, -28.2717) -> (-28.318, -29.0482) centre (-26.8691, -28.66) ccw
  line L33 (-25.4202, -28.2717) -> (-11.7739, -36.1504)
  circle A45 centre (64.5, -111.7173) radius 1.5
  arc A46 (39.8728, -10) -> (41.9941, -7.8787) centre (40.9335, -8.9393) ccw
  line L34 (39.8728, -10) -> (39.3155, -10)
  arc A47 (37.1941, -7.8787) -> (39.3155, -10) centre (38.2548, -8.9393) ccw
  line L35 (37.1941, -7.8787) -> (37.1941, 7.8787)
  arc A48 (39.3155, 10) -> (37.1941, 7.8787) centre (38.2548, 8.9393) ccw
  line L36 (39.3155, 10) -> (39.8728, 10)
  arc A49 (41.9941, 7.8787) -> (39.8728, 10) centre (40.9335, 8.9393) ccw
  line L37 (41.9941, 7.8787) -> (41.9941, -7.8787)
  circle A50 centre (-94.9024, -87.3758) radius 1.5
  circle A51 centre (-28.2185, -125.8758) radius 1.5
  circle A52 centre (64.5, 111.7173) radius 1.5
  arc A53 (-55.2202, 79.8868) -> (-55.9967, 76.9891) centre (-55.6084, 78.438) ccw
  line L38 (-55.2202, 79.8868) -> (-41.5739, 87.7655)
  arc A54 (-38.6762, 86.9891) -> (-41.5739, 87.7655) centre (-40.125, 87.3773) ccw
  line L39 (-38.6762, 86.9891) -> (-38.3975, 86.5064)
  arc A55 (-39.1739, 83.6086) -> (-38.3975, 86.5064) centre (-38.7857, 85.0575) ccw
  line L40 (-39.1739, 83.6086) -> (-52.8202, 75.7299)
  arc A56 (-55.718, 76.5064) -> (-52.8202, 75.7299) centre (-54.2691, 76.1181) ccw
  line L41 (-55.718, 76.5064) -> (-55.9967, 76.9891)
  circle A57 centre (123.1209, 38.5) radius 1.5
  circle A58 centre (45.4941, 42.5) radius 1.5
  circle A59 centre (-94.9024, 87.3758) radius 1.5
  arc A60 (94.6728, -10) -> (96.7941, -7.8787) centre (95.7335, -8.9393) ccw
  line L42 (94.6728, -10) -> (94.1155, -10)
  arc A61 (91.9941, -7.8787) -> (94.1155, -10) centre (93.0548, -8.9393) ccw
  line L43 (91.9941, -7.8787) -> (91.9941, 7.8787)
  arc A62 (94.1155, 10) -> (91.9941, 7.8787) centre (93.0548, 8.9393) ccw
  line L44 (94.1155, 10) -> (94.6728, 10)
  arc A63 (96.7941, 7.8787) -> (94.6728, 10) centre (95.7335, 8.9393) ccw
  line L45 (96.7941, 7.8787) -> (96.7941, -7.8787)
  circle A64 centre (45.4941, -42.5) radius 1.5
  line L46 (15.4941, -97) -> (41.8941, -97)
  arc A65 (45.5941, -100.7) -> (41.8941, -97) centre (41.8941, -100.7) ccw
  line L47 (45.5941, -100.7) -> (45.5941, -107.7)
  arc A66 (41.8941, -111.4) -> (45.5941, -107.7) centre (41.8941, -107.7) ccw
  line L48 (41.8941, -111.4) -> (15.4941, -111.4)
  arc A67 (11.7941, -107.7) -> (15.4941, -111.4) centre (15.4941, -107.7) ccw
  line L49 (11.7941, -107.7) -> (11.7941, -100.7)
  arc A68 (15.4941, -97) -> (11.7941, -100.7) centre (15.4941, -100.7) ccw
  line L50 (15.4941, 111.4) -> (41.8941, 111.4)
  arc A69 (45.5941, 107.7) -> (41.8941, 111.4) centre (41.8941, 107.7) ccw
  line L51 (45.5941, 107.7) -> (45.5941, 100.7)
  arc A70 (41.8941, 97) -> (45.5941, 100.7) centre (41.8941, 100.7) ccw
  line L52 (41.8941, 97) -> (15.4941, 97)
  arc A71 (11.7941, 100.7) -> (15.4941, 97) centre (15.4941, 100.7) ccw
  line L53 (11.7941, 100.7) -> (11.7941, 107.7)
  arc A72 (15.4941, 111.4) -> (11.7941, 107.7) centre (15.4941, 107.7) ccw
  circle A73 centre (97.2941, 62.4) radius 1.5
  circle A74 centre (97.2941, -62.4) radius 1.5
  circle A75 centre (64.2941, 62.4) radius 1.5
  circle A76 centre (64.2941, -62.4) radius 1.5
  arc A77 (65.7941, -100.26) -> (68.1301, -101.5054) centre (67.2941, -100.26) ccw
  line L54 (65.7941, -100.26) -> (65.7941, -74.3)
  arc A78 (67.2941, -72.8) -> (65.7941, -74.3) centre (67.2941, -74.3) ccw
  line L55 (67.2941, -72.8) -> (95.1844, -72.8)
  arc A79 (96.3668, -75.223) -> (95.1844, -72.8) centre (95.1844, -74.3) ccw
  arc A80 (68.1301, -101.5054) -> (96.3668, -75.223) centre (0, 0) ccw
  arc A81 (65.7941, 74.3) -> (67.2941, 72.8) centre (67.2941, 74.3) ccw
  line L56 (65.7941, 74.3) -> (65.7941, 100.26)
  arc A82 (68.1301, 101.5054) -> (65.7941, 100.26) centre (67.2941, 100.26) ccw
  arc A83 (96.3668, 75.223) -> (68.1301, 101.5054) centre (0, 0) ccw
  arc A84 (95.1844, 72.8) -> (96.3668, 75.223) centre (95.1844, 74.3) ccw
  line L57 (95.1844, 72.8) -> (67.2941, 72.8)
  line L58 (51.1728, 56) -> (18.4155, 56)
  arc A85 (16.2941, 58.1213) -> (18.4155, 56) centre (17.3548, 57.0607) ccw
  line L59 (16.2941, 58.1213) -> (16.2941, 59)
  line L60 (16.2941, 59) -> (13.9155, 59)
  arc A86 (11.7941, 61.1213) -> (13.9155, 59) centre (12.8548, 60.0607) ccw
  line L61 (11.7941, 61.1213) -> (11.7941, 86.8787)
  arc A87 (13.9155, 89) -> (11.7941, 86.8787) centre (12.8548, 87.9393) ccw
  line L62 (13.9155, 89) -> (16.2941, 89)
  line L63 (16.2941, 89) -> (16.2941, 89.8787)
  arc A88 (18.4155, 92) -> (16.2941, 89.8787) centre (17.3548, 90.9393) ccw
  line L64 (18.4155, 92) -> (51.1728, 92)
  arc A89 (53.2941, 89.8787) -> (51.1728, 92) centre (52.2335, 90.9393) ccw
  line L65 (53.2941, 89.8787) -> (53.2941, 89)
  line L66 (53.2941, 89) -> (55.6728, 89)
  arc A90 (57.7941, 86.8787) -> (55.6728, 89) centre (56.7335, 87.9393) ccw
  line L67 (57.7941, 86.8787) -> (57.7941, 61.1213)
  arc A91 (55.6728, 59) -> (57.7941, 61.1213) centre (56.7335, 60.0607) ccw
  line L68 (55.6728, 59) -> (53.2941, 59)
  line L69 (53.2941, 59) -> (53.2941, 58.1213)
  arc A92 (51.1728, 56) -> (53.2941, 58.1213) centre (52.2335, 57.0607) ccw
  line L70 (57.7941, -61.1213) -> (57.7941, -86.8787)
  arc A93 (55.6728, -89) -> (57.7941, -86.8787) centre (56.7335, -87.9393) ccw
  line L71 (55.6728, -89) -> (53.2941, -89)
  line L72 (53.2941, -89) -> (53.2941, -89.8787)
  arc A94 (51.1728, -92) -> (53.2941, -89.8787) centre (52.2335, -90.9393) ccw
  line L73 (51.1728, -92) -> (18.4155, -92)
  arc A95 (16.2941, -89.8787) -> (18.4155, -92) centre (17.3548, -90.9393) ccw
  line L74 (16.2941, -89.8787) -> (16.2941, -89)
  line L75 (16.2941, -89) -> (13.9155, -89)
  arc A96 (11.7941, -86.8787) -> (13.9155, -89) centre (12.8548, -87.9393) ccw
  line L76 (11.7941, -86.8787) -> (11.7941, -61.1213)
  arc A97 (13.9155, -59) -> (11.7941, -61.1213) centre (12.8548, -60.0607) ccw
  line L77 (13.9155, -59) -> (16.2941, -59)
  line L78 (16.2941, -59) -> (16.2941, -58.1213)
  arc A98 (18.4155, -56) -> (16.2941, -58.1213) centre (17.3548, -57.0607) ccw
  line L79 (18.4155, -56) -> (51.1728, -56)
  arc A99 (53.2941, -58.1213) -> (51.1728, -56) centre (52.2335, -57.0607) ccw
  line L80 (53.2941, -58.1213) -> (53.2941, -59)
  line L81 (53.2941, -59) -> (55.6728, -59)
  arc A100 (57.7941, -61.1213) -> (55.6728, -59) centre (56.7335, -60.0607) ccw
  circle A101 centre (0, 0) radius 3
  circle A102 centre (-100, 35.5) radius 1.5
  circle A103 centre (-53.2894, -35.5) radius 1.5
  circle A104 centre (-53.2894, 35.5) radius 1.5
  circle A105 centre (-100, -35.5) radius 1.5
  line L82 (53.2941, 59) -> (55.6728, 59)
  line L83 (53.2941, 58.1213) -> (53.2941, 59)
  arc A106 (51.1728, 56) -> (53.2941, 58.1213) centre (52.2335, 57.0607) ccw
  arc A107 (55.6728, 59) -> (57.7941, 61.1213) centre (56.7335, 60.0607) ccw
  arc A108 (57.7941, 86.8787) -> (55.6728, 89) centre (56.7335, 87.9393) ccw
  line L84 (53.2941, 89.8787) -> (53.2941, 89)
  arc A109 (53.2941, 89.8787) -> (51.1728, 92) centre (52.2335, 90.9393) ccw
  line L85 (53.2941, 89) -> (55.6728, 89)
  line L86 (16.2941, 92) -> (53.2941, 92)
  line L87 (57.7941, 89) -> (57.7941, 59)
  line L88 (11.7941, 61.1213) -> (11.7941, 86.8787)
  line L89 (16.2941, 59) -> (13.9155, 59)
  line L90 (13.9155, 89) -> (16.2941, 89)
  arc A110 (18.4155, 92) -> (16.2941, 89.8787) centre (17.3548, 90.9393) ccw
  arc A111 (13.9155, 89) -> (11.7941, 86.8787) centre (12.8548, 87.9393) ccw
  arc A112 (11.7941, 61.1213) -> (13.9155, 59) centre (12.8548, 60.0607) ccw
  arc A113 (16.2941, 58.1213) -> (18.4155, 56) centre (17.3548, 57.0607) ccw
  line L91 (51.1728, 56) -> (18.4155, 56)
  line L92 (16.2941, 56) -> (16.2941, 92)
  line L93 (51.1728, -92) -> (18.4155, -92)
  arc A114 (51.1728, -92) -> (53.2941, -89.8787) centre (52.2335, -90.9393) ccw
  arc A115 (55.6728, -89) -> (57.7941, -86.8787) centre (56.7335, -87.9393) ccw
  line L94 (53.2941, -89) -> (55.6728, -89)
  line L95 (57.7941, -61.1213) -> (57.7941, -86.8787)
  arc A116 (57.7941, -61.1213) -> (55.6728, -59) centre (56.7335, -60.0607) ccw
  line L96 (55.6728, -59) -> (53.2941, -59)
  arc A117 (53.2941, -58.1213) -> (51.1728, -56) centre (52.2335, -57.0607) ccw
  line L97 (18.4155, -56) -> (51.1728, -56)
  arc A118 (18.4155, -56) -> (16.2941, -58.1213) centre (17.3548, -57.0607) ccw
  line L98 (13.9155, -59) -> (16.2941, -59)
  arc A119 (13.9155, -59) -> (11.7941, -61.1213) centre (12.8548, -60.0607) ccw
  line L99 (11.7941, -61.1213) -> (11.7941, -86.8787)
  arc A120 (11.7941, -86.8787) -> (13.9155, -89) centre (12.8548, -87.9393) ccw
  arc A121 (16.2941, -89.8787) -> (18.4155, -92) centre (17.3548, -90.9393) ccw
  line L100 (13.9155, -89) -> (16.2941, -89)
  line L101 (16.2941, -89) -> (16.2941, -89.8787)
  line L102 (53.2941, -89.8787) -> (53.2941, -89)
  line L103 (53.2941, -58.1213) -> (53.2941, -59)
  line L104 (16.2941, -59) -> (16.2941, -58.1213)
extrude "Extrude16" add sketch "Sketch12" against normal blind 4.8 contours L58 A85 L59 L63 L64 A89 L65 L66 A90 L67 A91 L68 L69 A92 L82 L83 A106 A107 A108 L84 A109 L85 L86 L87 A113 L91 L92 | A85 A113 L92 | L60 A86 L61 A87 L62 L88 L89 L90 A111 A112 L92 | A91 A107 L87 | A88 A110 L92 | A90 A108 L87 | A88 L86 A110 | A89 A109 L86 | L70 A93 L71 L72 A94 L73 A95 L74 L75 A96 L76 A97 L77 L78 A98 L79 A99 L80 L81 A100 L93 A114 A115 L94 L95 A116 L96 A117 L97 A118 L98 A119 L99 A120 A121 L100 L101 L102 L103 L104